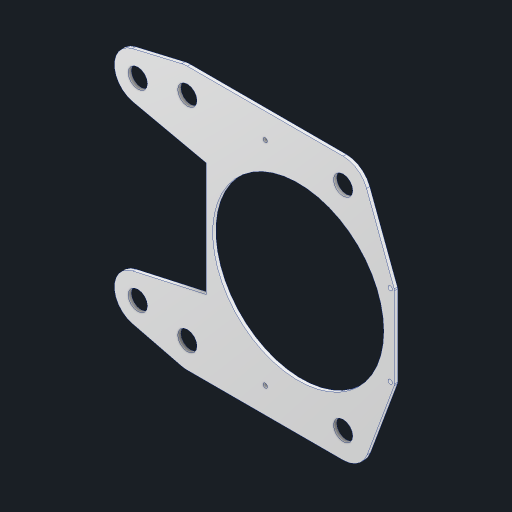
# Autodesk Inventor part: OUTK_002_ShotPlateReceptacle
Saved by Autodesk Inventor 2024.2 (Build 282272000, 272)
## iProperties
Created: 2024-11-24
Part Number: OUTK_002_ShotPlateReceptacle
Material: Aluminum 6061
Document SubType Name: Modeling
Designer: Bryan
Density: 2.7 g/cm^3
Appearance: Aluminum - Flat
Author: Bryan
Autodesk Inventor part; units mm, degrees
ref_plane "YZ Plane" through (0, 0, 0) normal (1, 0, 0) x (0, 1, 0)
ref_plane "XZ Plane" through (0, 0, 0) normal (0, 1, 0) x (-1, 0, 0)
ref_plane "XY Plane" through (0, 0, 0) normal (0, 0, 1) x (1, 0, 0)
sketch "Sketch1" plane through (0, 0, 0) normal (0, 0, 1) x (1, 0, 0)
  circle A0 centre (0, 142.875) radius 63.5 construction
  circle A1 centre (0, 142.875) radius 25.4 construction
  circle A2 centre (0, -142.875) radius 25.4 construction
  circle A3 centre (0, -142.875) radius 63.5 construction
  line L0 (0, 79.375) -> (0, 79.375) construction
  line L1 (0, -79.375) -> (0, -79.375) construction
  line L2 (0, 0) -> (228.6, 0) construction
  line L3 (0, 142.875) -> (304.8, 142.875) construction
  line L4 (304.8, 142.875) -> (304.8, -142.875) construction
  line L5 (304.8, -142.875) -> (0, -142.875) construction
  circle A4 centre (228.6, 0) radius 127 construction
  circle A5 centre (0, 142.875) radius 14.2875
  circle A6 centre (0, -142.875) radius 14.2875
  circle A7 centre (0, 142.875) radius 34.925 construction
  circle A8 centre (0, -142.875) radius 34.925 construction
  circle A9 centre (73.5068, -157.7975) radius 22.225 construction
  circle A10 centre (73.5068, -157.7975) radius 33.3375 construction
  circle A11 centre (73.5068, -157.7975) radius 11.1125 construction
  line L6 (73.5068, -146.685) -> (73.5068, -135.5725) construction
  line L7 (73.5068, -124.46) -> (73.5068, -135.5725) construction
  circle A12 centre (304.8, -157.7975) radius 33.3375 construction
  circle A13 centre (304.8, -157.7975) radius 14.2875
  circle A14 centre (374.65, 60.0642) radius 6.35 construction
  circle A15 centre (374.65, -60.0642) radius 6.35 construction
  line L8 (304.8, 157.7975) -> (374.65, 60.0642) construction
  line L9 (374.65, 60.0642) -> (374.65, -60.0642) construction
  line L10 (374.65, -60.0642) -> (304.8, -157.7975) construction
  line L11 (-118.745, 84.5312) -> (101.6, 84.5312) construction
  line L12 (101.6, 84.5312) -> (101.6, -84.5312) construction
  line L13 (101.6, -84.5312) -> (-118.745, -84.5312) construction
  line L14 (-118.745, -84.5312) -> (-118.745, 84.5312) construction
  line L15 (0, 142.875) -> (0, 84.5312) construction
  line L16 (0, -84.5312) -> (0, -142.875) construction
  circle A16 centre (73.5068, -157.7975) radius 14.2875
  line L17 (73.5068, -124.46) -> (304.8, -124.46) construction
  circle A17 centre (73.5068, 0) radius 127 construction
  circle A18 centre (0, 0) radius 127 construction
  circle A19 centre (0, 142.875) radius 6.35 construction
  circle A20 centre (73.5068, 157.7975) radius 33.3375 construction
  circle A21 centre (304.8, 157.7975) radius 33.3375 construction
  circle A22 centre (304.8, 157.7975) radius 14.2875
  circle A23 centre (73.5068, 157.7975) radius 14.2875
  circle A24 centre (73.5068, 157.7975) radius 37.1475 construction
  circle A25 centre (304.8, 157.7975) radius 37.1475 construction
  circle A26 centre (304.8, -157.7975) radius 38.1 construction
  circle A27 centre (73.5068, -157.7975) radius 38.1 construction
  line L18 (-7.9595, 176.8809) -> (65.0408, 193.9674)
  line L19 (73.5068, 194.945) -> (304.8, 194.945)
  line L20 (339.5497, 170.9273) -> (380.5901, 62.3086)
  line L21 (381, 60.0642) -> (381, -60.0642)
  line L22 (64.3531, -194.7815) -> (-8.3909, -176.777)
  line L23 (220.4162, -245.7989) -> (237.7908, -293.5353) construction
  line L24 (237.7908, -293.5353) -> (381, -241.4114) construction
  line L25 (381, -241.4114) -> (363.6254, -193.675) construction
  line L26 (363.6254, -193.675) -> (220.4162, -245.7989) construction
  line L27 (-7.573, -108.7809) -> (101.6, -84.5312)
  line L28 (-7.573, 108.7809) -> (101.6, 84.5312)
  line L29 (101.6, 84.5312) -> (101.6, -84.5312)
  circle A28 centre (238.125, 0) radius 127
  line L30 (101.6, 0) -> (111.125, 0)
  line L31 (374.65, 0) -> (365.125, 0)
  circle A29 centre (220.4162, -245.7989) radius 3.2512 construction
  circle A30 centre (268.1526, -228.4242) radius 3.2512 construction
  circle A31 centre (315.889, -211.0496) radius 3.2512 construction
  circle A32 centre (363.6254, -193.675) radius 3.2512 construction
  circle A33 centre (237.7908, -293.5353) radius 3.2512 construction
  circle A34 centre (285.5272, -276.1606) radius 3.2512 construction
  circle A35 centre (333.2636, -258.786) radius 3.2512 construction
  circle A36 centre (381, -241.4114) radius 3.2512 construction
  line L32 (73.5068, -195.8975) -> (304.8, -195.8975)
  line L33 (380.6084, -62.2597) -> (340.5502, -170.9708)
  arc A37 (-7.9595, 176.8809) -> (-7.573, 108.7809) centre (0, 142.875) ccw
  arc A38 (73.5068, 194.945) -> (65.0408, 193.9674) centre (73.5068, 157.7975) ccw
  arc A39 (339.5497, 170.9273) -> (304.8, 194.945) centre (304.8, 157.7975) ccw
  arc A40 (381, 60.0642) -> (380.5901, 62.3086) centre (374.65, 60.0642) ccw
  arc A41 (380.6084, -62.2597) -> (381, -60.0642) centre (374.65, -60.0642) ccw
  arc A42 (304.8, -195.8975) -> (340.5502, -170.9708) centre (304.8, -157.7975) ccw
  arc A43 (64.3531, -194.7815) -> (73.5068, -195.8975) centre (73.5068, -157.7975) ccw
  arc A44 (-7.573, -108.7809) -> (-8.3909, -176.777) centre (0, -142.875) ccw
  circle A45 centre (374.65, 60.0642) radius 3.2512
  circle A46 centre (374.65, -60.0642) radius 3.2512
  circle A47 centre (189.1534, 157.7975) radius 3.2512
  line L34 (73.5068, 157.7975) -> (189.1534, 157.7975) construction
  line L35 (189.1534, 157.7975) -> (304.8, 157.7975) construction
  circle A48 centre (189.1534, -157.7975) radius 3.2512
  point P0 (0, 117.475)
  point P1 (0, -117.475)
  point P2 (304.8, 0)
  point P3 (228.6, -127)
  point P4 (228.6, -127)
  point P5 (355.6, 0)
  point P6 (0, 127)
  point P7 (0, 117.475)
  point P8 (0, 136.525)
  dimension "d1" = 50.8
  dimension "d16" = 44.45
  dimension "d20" = 22.225
  dimension "d33" = 12.7
  dimension "d0" = 127
  dimension "d3" = 285.75
  dimension "d4" = 254
  dimension "d6" = 158.75
  dimension "d7" = 234.95
  dimension "d11" = 28.575
  dimension "d12" = 28.575
  dimension "d13" = 69.85
  dimension "d14" = 69.85
  dimension "d19" = 76.2
  dimension "d22" = 304.8
  dimension "d24" = 28.575
  dimension "d26" = 12.7
  dimension "d27" = 12.7
  dimension "d28" = 19.05
  dimension "d29" = 220.345
  dimension "d30" = 169.0624
  dimension "d31" = 2.54
  dimension "d32" = 75.0062
  dimension "d34" = 9.525
  dimension "d35" = 19.05
  dimension "d37" = 3.81
  dimension "d38" = 3.81
  dimension "d39" = 4.7625
  dimension "d40" = 4.7625
  dimension "d43" = 20
  dimension "d44" = 6.5024
  dimension "d47" = 50.8
  dimension "d50" = 50.8
  dimension "d53" = 50.8
  dimension "d56" = 6.5024
  dimension "d57" = 6.5024
  dimension "d58" = 6.5024
  constraints: 72 end point, 41 centre point, 41 point on circle, 24 tangent, 21 coincident, 16 vertical alignment, 11 horizontal, 7 perpendicular, 7 point on line, 6 concentric, 6 equal length, 6 symmetric about line, 4 equal radius, 4 vertical, 3 horizontal alignment, 3 midpoint, 2 parallel, 41 other
  measures "d0" diameter of A0
  measures "d3" distance between parallel lines of L5 L3
  measures "d4" diameter of A4
  measures "d6" distance of L1.start L0.start
  measures "d7" distance of point (0, -117.475) point (0, 117.475)
  measures "d11" diameter of A5
  measures "d12" diameter of A6
  measures "d13" diameter of A7
  measures "d14" diameter of A8
  measures "d19" distance of point (304.8, 0) L2.end
  measures "d22" distance of L3.end A0.centre
  measures "d24" diameter of A13
  measures "d26" diameter of A14
  measures "d27" diameter of A15
  measures "d28" distance from line of L9 point (355.6, 0)
  measures "d29" distance of L12.end L13.end
  measures "d30" distance of L11.end L12.end
  measures "d31" distance from line of L17 A4.start
  measures "d32" distance of point (73.507, -157.798) point (0, -142.875)
  measures "d34" distance of point (0, 117.475) point (0, 127)
  measures "d35" distance of point (0, 117.475) point (0, 136.525)
  measures "d37" radial gap between concentric circles of A20 A24
  measures "d38" radial gap between concentric circles of A21 A25
  measures "d43" angle of L26 L5
  measures "d44" diameter of A29
  measures "d47" distance of A29.centre A30.centre
  measures "d50" distance of A29.centre A33.centre
  measures "d53" distance from line of L25.end L5
  measures "d56" diameter of A45
  measures "d57" diameter of A46
  measures "d58" diameter of A47
extrude "Extrusion1" add sketch "Sketch1" along normal mid plane 4.7625
sketch "Sketch2" plane through (0, 0, -2.3813) normal (0, 0, -1) x (-1, 0, 0)
  line L0 (7.573, -108.7809) -> (-101.6, -84.5312) projected
  line L1 (-101.6, -84.5312) -> (-101.6, 84.5312) projected
  line L2 (-101.6, 84.5312) -> (7.573, 108.7809) projected
  arc A0 (7.573, 108.7809) -> (7.9595, 176.8809) centre (0, 142.875) ccw projected
  line L3 (7.9595, 176.8809) -> (-65.0408, 193.9674) projected
  arc A1 (-65.0408, 193.9674) -> (-73.5068, 194.945) centre (-73.5068, 157.7975) ccw projected
  line L4 (-73.5068, 194.945) -> (-304.8, 194.945) projected
  arc A2 (-304.8, 194.945) -> (-339.5497, 170.9273) centre (-304.8, 157.7975) ccw projected
  line L5 (-339.5497, 170.9273) -> (-380.5901, 62.3086) projected
  arc A3 (-380.5901, 62.3086) -> (-381, 60.0642) centre (-374.65, 60.0642) ccw projected
  line L6 (-381, 60.0642) -> (-381, -60.0642) projected
  arc A4 (-381, -60.0642) -> (-380.6084, -62.2597) centre (-374.65, -60.0642) ccw projected
  line L7 (-380.6084, -62.2597) -> (-340.5502, -170.9708) projected
  arc A5 (-340.5502, -170.9708) -> (-304.8, -195.8975) centre (-304.8, -157.7975) ccw projected
  line L8 (-304.8, -195.8975) -> (-73.5068, -195.8975) projected
  arc A6 (-73.5068, -195.8975) -> (-64.3531, -194.7815) centre (-73.5068, -157.7975) ccw projected
  line L9 (-64.3531, -194.7815) -> (8.3909, -176.777) projected
  arc A7 (8.3909, -176.777) -> (7.573, -108.7809) centre (0, -142.875) ccw projected
  circle A8 centre (-238.125, 0) radius 127 projected
  circle A9 centre (-73.5068, -157.7975) radius 14.2875 projected
  circle A10 centre (-73.5068, 157.7975) radius 14.2875 projected
  circle A11 centre (-189.1534, 157.7975) radius 3.2512 projected
  circle A12 centre (-189.1534, -157.7975) radius 3.2512 projected
  circle A13 centre (-374.65, -60.0642) radius 3.2512 projected
  circle A14 centre (-374.65, 60.0642) radius 3.2512 projected
  circle A15 centre (-304.8, 157.7975) radius 14.2875 projected
  circle A16 centre (-304.8, -157.7975) radius 14.2875 projected
  circle A17 centre (0, -142.875) radius 14.2875 projected
  circle A18 centre (0, 142.875) radius 14.2875 projected
  line L10 (-106.3625, -88.3519) -> (6.5404, -113.4301)
  arc A19 (7.2467, -172.154) -> (6.5404, -113.4301) centre (0, -142.875) ccw
  line L11 (7.2467, -172.154) -> (-65.4973, -190.1585)
  arc A20 (-73.5068, -191.135) -> (-65.4973, -190.1585) centre (-73.5068, -157.7975) ccw
  line L12 (-73.5068, -191.135) -> (-304.8, -191.135)
  arc A21 (-336.0814, -169.3242) -> (-304.8, -191.135) centre (-304.8, -157.7975) ccw
  line L13 (-336.0814, -169.3242) -> (-376.1396, -60.6131)
  arc A22 (-376.2375, -60.0642) -> (-376.1396, -60.6131) centre (-374.65, -60.0642) ccw
  line L14 (-376.2375, -60.0642) -> (-376.2375, 60.0642)
  arc A23 (-376.135, 60.6253) -> (-376.2375, 60.0642) centre (-374.65, 60.0642) ccw
  line L15 (-376.135, 60.6253) -> (-335.0947, 169.244)
  arc A24 (-304.8, 190.1825) -> (-335.0947, 169.244) centre (-304.8, 157.7975) ccw
  line L16 (-304.8, 190.1825) -> (-73.5068, 190.1825)
  arc A25 (-66.1262, 189.3303) -> (-73.5068, 190.1825) centre (-73.5068, 157.7975) ccw
  line L17 (-66.1262, 189.3303) -> (6.8741, 172.2438)
  arc A26 (6.5404, 113.4301) -> (6.8741, 172.2438) centre (0, 142.875) ccw
  line L18 (6.5404, 113.4301) -> (-106.3625, 88.3519)
  line L19 (-106.3625, 88.3519) -> (-106.3625, -88.3519)
  circle A27 centre (-238.125, 0) radius 133.35
  circle A28 centre (-73.5068, 157.7975) radius 19.05
  circle A29 centre (0, 142.875) radius 19.05
  circle A30 centre (-189.1534, 157.7975) radius 8.0137
  circle A31 centre (-304.8, 157.7975) radius 19.05
  circle A32 centre (-374.65, 60.0642) radius 8.0137
  circle A33 centre (-374.65, -60.0642) radius 8.0137
  circle A34 centre (-304.8, -157.7975) radius 19.05
  circle A35 centre (-189.1534, -157.7975) radius 8.0137
  circle A36 centre (-73.5068, -157.7975) radius 19.05
  circle A37 centre (0, -142.875) radius 19.05
  line L20 (0, -142.875) -> (-73.5068, -157.7975)
  line L21 (-73.5068, -157.7975) -> (-68.896, -195.6175)
  line L22 (-73.5068, -157.7975) -> (-101.6, -84.5312)
  line L23 (-73.5068, -157.7975) -> (-189.1534, -157.7975)
  line L24 (-189.1534, -157.7975) -> (-189.1534, -195.8975)
  line L25 (-189.1534, -157.7975) -> (-304.8, -157.7975)
  line L26 (-304.8, -157.7975) -> (-326.5911, -189.0506)
  line L27 (-101.6, -84.5312) -> (-238.125, 0)
  line L28 (-238.125, 0) -> (-189.1534, -157.7975)
  line L29 (-304.8, -157.7975) -> (-238.125, 0)
  line L30 (-238.125, 0) -> (-374.65, -60.0642)
  line L31 (-238.125, 0) -> (-374.65, 60.0642)
  line L32 (-374.65, 60.0642) -> (-304.8, 157.7975)
  line L33 (-304.8, 157.7975) -> (-189.1534, 157.7975)
  line L34 (-189.1534, 157.7975) -> (-73.5068, 157.7975)
  line L35 (-73.5068, 157.7975) -> (0, 142.875)
  line L36 (-101.6, -84.5312) -> (-189.1534, -157.7975)
  line L37 (-304.8, -157.7975) -> (-374.65, -60.0642)
  line L38 (-101.6, 84.5312) -> (-73.5068, 157.7975)
  line L39 (-101.6, 84.5312) -> (-189.1534, 157.7975)
  line L40 (-101.6, 84.5312) -> (-238.125, 0)
  line L41 (-238.125, 0) -> (-189.1534, 157.7975)
  line L42 (-238.125, 0) -> (-304.8, 157.7975)
  line L43 (-4.7625, -138.9822) -> (-74.4543, -153.1302)
  line L44 (-69.06, -156.0924) -> (-97.1532, -82.8261)
  line L45 (0, -142.875) -> (0, -111.9774)
  line L46 (-4.7625, -110.9195) -> (-4.7625, -138.9822)
  line L47 (0, 142.875) -> (0, 111.9774)
  line L48 (-97.1532, 82.8261) -> (-69.06, 156.0924)
  line L49 (-106.0468, 86.2363) -> (-77.9536, 159.5026)
  line L50 (-189.1534, 153.035) -> (-73.5068, 153.035)
  line L51 (-98.5436, 88.1836) -> (-186.097, 161.4499)
  line L52 (-104.1071, 88.5804) -> (-240.6321, 4.0492)
  line L53 (-104.6564, 80.8788) -> (-192.2098, 154.1451)
  line L54 (-233.5765, -1.4116) -> (-184.6049, 156.3859)
  line L55 (-242.6735, 1.4116) -> (-193.7019, 159.2091)
  line L56 (-304.8, 153.035) -> (-189.1534, 153.035)
  line L57 (-233.738, 1.8536) -> (-300.413, 159.6511)
  line L58 (-242.512, -1.8536) -> (-309.187, 155.9439)
  line L59 (-300.9254, 155.0283) -> (-367.3675, 62.0633)
  line L60 (-367.3675, 62.0633) -> (-236.2071, 4.3593)
  line L61 (-240.0429, -4.3593) -> (-381.9325, 58.0651)
  line L62 (-381.9325, 58.0651) -> (-308.6746, 160.5667)
  line L63 (-240.0429, 4.3593) -> (-381.9325, -58.0651)
  line L64 (-381.9325, -58.0651) -> (-308.6746, -160.5667)
  line L65 (-236.2071, -4.3593) -> (-367.3675, -62.0633)
  line L66 (-367.3675, -62.0633) -> (-300.9254, -155.0283)
  line L67 (-309.187, -155.9439) -> (-242.512, 1.8536)
  line L68 (-242.6735, -1.4116) -> (-193.7019, -159.2091)
  line L69 (-233.5765, 1.4116) -> (-184.6049, -156.3859)
  line L70 (-300.413, -159.6511) -> (-233.738, -1.8536)
  line L71 (-104.1071, -88.5804) -> (-240.6321, -4.0492)
  line L72 (-99.0929, -80.482) -> (-235.6179, 4.0492)
  line L73 (-99.0929, 80.482) -> (-235.6179, -4.0492)
  line L74 (-77.9536, -159.5026) -> (-106.0468, -86.2363)
  line L75 (-106.3701, -82.3128) -> (-193.9235, -155.5791)
  line L76 (-98.5436, -88.1836) -> (-186.097, -161.4499)
  line L77 (-73.5068, -153.035) -> (-189.1534, -153.035)
  line L78 (-189.1534, -153.035) -> (-304.8, -153.035)
  line L79 (-74.4543, 153.1302) -> (-4.7625, 138.9822)
  line L80 (-4.7625, 138.9822) -> (-4.7625, 110.9195)
  arc A38 (-376.2375, -6.35) -> (-371.3291, -6.2352) centre (-373.782, -6.35) ccw
  arc A39 (-371.3291, 6.2352) -> (-376.2375, 6.35) centre (-373.782, 6.35) ccw
  line L81 (-238.125, 0) -> (-365.125, 0)
  point P0 (0, 0)
  dimension "d59" = 4.7625
  dimension "d60" = 6.35
  dimension "d61" = 4.7625
  dimension "d62" = 4.7625
  dimension "d63" = 4.7625
  dimension "d64" = 4.7625
  dimension "d65" = 4.7625
  dimension "d66" = 4.7625
  dimension "d67" = 4.7625
  dimension "d68" = 4.7625
  dimension "d69" = 4.7625
  dimension "d70" = 4.7625
  dimension "d71" = 4.7625
  dimension "d72" = 4.7625
  dimension "d73" = 4.7625
  dimension "d75" = 4.7625
  dimension "d76" = 4.7625
  dimension "d77" = 4.7625
  dimension "d78" = 4.7625
  dimension "d79" = 4.7625
  dimension "d80" = 4.7625
  dimension "d81" = 4.7625
  dimension "d82" = 4.7625
  dimension "d83" = 4.7625
  dimension "d84" = 4.7625
  dimension "d85" = 4.7625
  dimension "d86" = 4.7625
  dimension "d87" = 4.7625
  dimension "d88" = 4.7625
  dimension "d89" = 4.7625
  dimension "d90" = 4.7625
  dimension "d91" = 4.7625
  dimension "d92" = 4.7625
  dimension "d93" = 4.7625
  dimension "d94" = 4.7625
  dimension "d95" = 4.7625
  dimension "d96" = 4.7625
  dimension "d97" = 4.7625
  dimension "d98" = 4.7625
  dimension "d99" = 4.7625
  dimension "d100" = 4.7625
  dimension "d101" = 4.7625
  dimension "d102" = 4.7625
  dimension "d103" = 4.7625
  dimension "d104" = 12.7
  constraints: 144 end point, 25 parallel, 24 point on circle, 21 centre point, 6 point on line, 5 horizontal, 4 tangent, 2 vertical, 1 horizontal alignment, 1 midpoint, 1 symmetric about line, 22 other
  measures "d59" distance between parallel lines of L0 L10
  measures "d61" radial gap between concentric circles of A10 A28
  measures "d62" radial gap between concentric circles of A18 A29
  measures "d63" radial gap between concentric circles of A11 A30
  measures "d64" radial gap between concentric circles of A15 A31
  measures "d65" radial gap between concentric circles of A14 A32
  measures "d66" radial gap between concentric circles of A13 A33
  measures "d67" radial gap between concentric circles of A16 A34
  measures "d68" radial gap between concentric circles of A12 A35
  measures "d69" radial gap between concentric circles of A9 A36
  measures "d70" radial gap between concentric circles of A17 A37
  measures "d71" distance between parallel lines of L20 L43
  measures "d72" distance between parallel lines of L22 L44
  measures "d73" distance between parallel lines of L45 L46
  measures "d75" distance between parallel lines of L38 L48
  measures "d76" distance between parallel lines of L38 L49
  measures "d77" distance between parallel lines of L34 L50
  measures "d78" distance between parallel lines of L39 L51
  measures "d79" distance between parallel lines of L40 L52
  measures "d80" distance between parallel lines of L39 L53
  measures "d81" distance between parallel lines of L41 L54
  measures "d82" distance between parallel lines of L41 L55
  measures "d83" distance between parallel lines of L33 L56
  measures "d84" distance between parallel lines of L42 L57
  measures "d85" distance between parallel lines of L42 L58
  measures "d86" distance between parallel lines of L32 L59
  measures "d87" distance between parallel lines of L31 L61
  measures "d88" distance between parallel lines of L30 L63
  measures "d89" distance between parallel lines of L30 L65
  measures "d90" distance between parallel lines of L29 L67
  measures "d91" distance between parallel lines of L28 L68
  measures "d92" distance between parallel lines of L28 L69
  measures "d93" distance between parallel lines of L29 L70
  measures "d94" distance between parallel lines of L27 L71
  measures "d95" distance between parallel lines of L27 L72
  measures "d96" distance between parallel lines of L40 L73
  measures "d97" distance between parallel lines of L22 L74
  measures "d98" distance between parallel lines of L36 L75
  measures "d99" distance between parallel lines of L36 L76
  measures "d100" distance between parallel lines of L23 L77
  measures "d101" distance between parallel lines of L25 L78
  measures "d102" distance between parallel lines of L35 L79
  measures "d103" distance between parallel lines of L47 L80
  measures "d104" distance of A39.centre A38.centre
body "Solid1"
